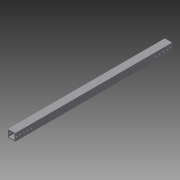
# Autodesk Inventor part: Roller Sidways 21.375 in Segment (1)
Saved by Autodesk Inventor 2014 (Build 180170000, 170)
## iProperties
Created: 2014-02-24
Part Number: Roller Sidways 21.375 in Segment (1)
Material: Generic
Document SubType Name: Modeling
Designer: Michael
Density: 1 g/cm^3
Appearance: Default
Author: Michael
Autodesk Inventor part; units mm, degrees
ref_plane "YZ Plane" through (0, 0, 0) normal (1, 0, 0) x (0, 1, 0)
ref_plane "XZ Plane" through (0, 0, 0) normal (0, 1, 0) x (-1, 0, 0)
ref_plane "XY Plane" through (0, 0, 0) normal (0, 0, 1) x (1, 0, 0)
sketch "Sketch1" plane through (0, 0, 0) normal (0, 0, 1) x (1, 0, 0)
  line L0 (0, 0) -> (25.4, 0)
  line L1 (25.4, 0) -> (25.4, 25.4)
  line L2 (25.4, 25.4) -> (0, 25.4)
  line L3 (0, 25.4) -> (0, 0)
  line L4 (3.175, 22.225) -> (22.225, 22.225)
  line L5 (22.225, 22.225) -> (22.225, 3.175)
  line L6 (22.225, 3.175) -> (3.175, 3.175)
  line L7 (3.175, 3.175) -> (3.175, 22.225)
  dimension "d0" = 25.4
  dimension "d1" = 25.4
  dimension "d2" = 3.175
  constraints: 16 end point, 4 parallel, 2 perpendicular, 1 horizontal, 3 other
  measures "d0" distance of L2.end L1.end
  measures "d1" distance of L1.end L0.end
  measures "d2" distance between parallel lines of L2 L4
extrude "Extrusion1" add sketch "Sketch1" along normal blind 542.925
sketch "Sketch2" plane through (25.4, 0, 0) normal (1, 0, 0) x (0, 0, -1)
  line L0 (0, 25.4) -> (-542.925, 25.4) projected
  line L1 (-542.925, 0) -> (-542.925, 25.4) projected
  line L2 (0, 0) -> (-542.925, 0) projected
  circle A0 centre (-538.1625, 12.7) radius 2.0701
  circle A1 centre (-525.4625, 12.7) radius 2.0701
  circle A2 centre (-512.7625, 12.7) radius 2.0701
  circle A3 centre (-500.0625, 12.7) radius 2.0701
  circle A4 centre (-487.3625, 12.7) radius 2.0701
  line L3 (-271.4625, 25.4) -> (-271.4625, 0) construction
  circle A5 centre (-4.7625, 12.7) radius 2.0701
  circle A6 centre (-17.4625, 12.7) radius 2.0701
  circle A7 centre (-30.1625, 12.7) radius 2.0701
  circle A8 centre (-42.8625, 12.7) radius 2.0701
  circle A9 centre (-55.5625, 12.7) radius 2.0701
  dimension "d5" = 4.1402
  dimension "d6" = 4.7625
  dimension "d7" = 12.7
  dimension "d10" = 12.7
  constraints: 10 centre point, 5 symmetric about line, 2 end point, 2 midpoint, 1 horizontal, 13 other
  measures "d5" diameter of A0
  measures "d6" distance from line of L1 A0.centre
  measures "d7" distance from line of L2 A0.centre
  measures "d10" distance of A0.centre A1.centre
extrude "Extrusion2" cut sketch "Sketch2" against normal blind 593.725
body "Solid1"
